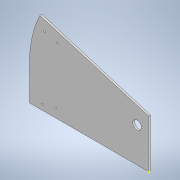
# Autodesk Inventor part: TurretPanel
Saved by Autodesk Inventor 2022 (Build 260153000, 153)
## iProperties
Created: 2022-01-18
Part Number: TurretPanel
Material: Generic
Document SubType Name: Modeling
Designer: tagaz
Density: 1 g/cm^3
Appearance: Default
Author: tagaz
Autodesk Inventor part; units mm, degrees
ref_plane "YZ Plane" through (0, 0, 0) normal (1, 0, 0) x (0, 1, 0)
ref_plane "XZ Plane" through (0, 0, 0) normal (0, 1, 0) x (-1, 0, 0)
ref_plane "XY Plane" through (0, 0, 0) normal (0, 0, 1) x (1, 0, 0)
sketch "Sketch1" plane through (0, 0, 0) normal (0, 0, 1) x (1, 0, 0)
  line L0 (0, 0) -> (-393.7, 0)
  line L1 (-393.7, 0) -> (-393.7, 114.3)
  line L2 (0, 203.2) -> (0, 0)
  circle A0 centre (-38.1, 114.3) radius 50.8 construction
  circle A1 centre (-38.1, 114.3) radius 6.35 construction
  circle A2 centre (-38.1, 114.3) radius 14.2875
  line L3 (-38.1, 114.3) -> (-38.1, 165.1)
  arc A3 (-384.7802, 193.4467) -> (-393.7, 114.3) centre (-38.1, 114.3) ccw
  arc A4 (-338.2351, 305.01) -> (-393.6892, 111.5268) centre (-38.1, 114.3) ccw
  circle A5 centre (-38.1, 114.3) radius 282.575 construction
  circle A6 centre (-38.1, 114.3) radius 327.025 construction
  circle A7 centre (-38.1, 114.3) radius 304.8 construction
  arc A8 (-372.5283, 214.9641) -> (-378.0555, 34.2635) centre (-38.1, 114.3) ccw
  arc A9 (-287.4011, 189.3405) -> (-291.5214, 54.6365) centre (-38.1, 114.3) ccw
  arc A10 (-287.4011, 189.3405) -> (-372.5283, 214.9641) centre (-329.9647, 202.1523) ccw construction
  arc A11 (-378.0555, 34.2635) -> (-291.5214, 54.6365) centre (-334.7884, 44.45) ccw construction
  line L4 (-38.1, 114.3) -> (-329.9647, 202.1523) construction
  line L5 (-38.1, 114.3) -> (-334.7884, 44.45) construction
  circle A12 centre (-301.445, 216.7599) radius 3.175
  circle A13 centre (-344.1211, 229.6101) radius 3.175
  circle A14 centre (-350.5965, 17.9088) radius 3.175
  circle A15 centre (-307.2148, 28.1267) radius 3.175
  line L6 (0, 203.2) -> (-338.2351, 305.01)
  point P0 (-356.4219, 39.3568)
  point P1 (-313.1549, 49.5432)
  point P2 (-308.6829, 195.7464)
  point P3 (-351.2465, 208.5582)
  point P4 (-384.7802, 193.4467)
  dimension "d2" = 101.6
  dimension "d38" = 609.6
  dimension "d3" = 12.7
  dimension "d4" = 28.575
  dimension "d5" = 114.3
  dimension "d22" = 114.3
  dimension "d24" = 38.1
  dimension "d25" = 304.8
  dimension "d30" = 565.15
  dimension "d31" = 654.05
  dimension "d39" = 30
  dimension "d40" = 88.9
  dimension "d43" = 6.35
  dimension "d44" = 6.35
  dimension "d45" = 6.35
  dimension "d46" = 6.35
  dimension "d47" = 22.225
  dimension "d48" = 22.225
  dimension "d49" = 22.225
  dimension "d50" = 22.225
  dimension "d51" = 203.2
  constraints: 20 point on circle, 14 centre point, 14 end point, 7 coincident, 5 tangent, 4 point on line, 2 parallel, 1 concentric, 1 horizontal, 1 horizontal alignment, 1 perpendicular, 1 vertical, 1 vertical alignment, 5 other
  measures "d3" diameter of A1
  measures "d4" diameter of A2
  measures "d5" distance from line of L0 A3.centre
  measures "d22" distance of L0.end L1.end
  measures "d24" distance from line of L2 A3.centre
  measures "d30" diameter of A5
  measures "d31" diameter of A6
  measures "d39" angle of L4 L5
  measures "d40" diameter of A10
  measures "d43" diameter of A12
  measures "d44" diameter of A13
  measures "d45" diameter of A14
  measures "d46" diameter of A15
  measures "d47" distance of point (-308.683, 195.746) A12.centre
  measures "d48" distance of point (-351.247, 208.558) A13.centre
  measures "d49" distance of point (-313.155, 49.543) A15.centre
  measures "d50" distance of point (-356.422, 39.357) A14.centre
  measures "d51" distance of L2.start L0.start
extrude "Extrusion1" add sketch "Sketch1" along normal blind 6.35
sketch "Sketch2" plane through (0, 0, 6.35) normal (0, 0, 1) x (1, 0, 0)
  point P0 (0, 0)
sketch "Sketch3" plane through (0, 0, 6.35) normal (0, 0, 1) x (1, 0, 0)
  line L0 (0, 0) -> (0, 203.2) projected
  line L1 (0, 203.2) -> (-338.2351, 305.01) projected
  arc A0 (-338.2351, 305.01) -> (-393.7, 114.3) centre (-38.1, 114.3) ccw projected
  line L2 (-393.7, 114.3) -> (-393.7, 0) projected
  line L3 (-393.7, 0) -> (0, 0) projected
  circle A1 centre (-38.1, 114.3) radius 14.2875 projected
  circle A2 centre (-350.5965, 17.9088) radius 3.175 projected
  circle A3 centre (-307.2148, 28.1267) radius 3.175 projected
  circle A4 centre (-344.1211, 229.6101) radius 3.175 projected
  circle A5 centre (-301.445, 216.7599) radius 3.175 projected
  line L4 (0, 0) -> (0, 203.2) projected
  line L5 (0, 159.181) -> (-359.1138, 267.2755)
  dimension "d52" = 31.75
  constraints: 2 end point, 1 parallel, 1 point on circle, 1 point on line
  measures "d52" distance from line of A5.centre L5
extrude "Extrusion2" cut sketch "Sketch3" against normal blind 25.4 contours L5 A0 L1 L0
body "Solid1"
